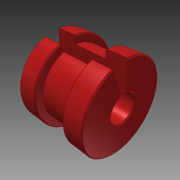
# Autodesk Inventor part: coupling_tie
Saved by Autodesk Inventor 2014 (Build 180170000, 170)
## iProperties
Created: 2014-01-25
Part Number: coupling_tie
Material: ABS Plastic
Document SubType Name: Modeling
Designer: buben
Density: 1.06 g/cm^3
Appearance: Light Red
Author: buben
Autodesk Inventor part; units mm, degrees
ref_plane "YZ Plane" through (0, 0, 0) normal (1, 0, 0) x (0, 1, 0)
ref_plane "XZ Plane" through (0, 0, 0) normal (0, 1, 0) x (-1, 0, 0)
ref_plane "XY Plane" through (0, 0, 0) normal (0, 0, 1) x (1, 0, 0)
sketch "Sketch1" plane through (0, 0, 0) normal (0, 1, 0) x (-1, 0, 0)
  line L0 (-9, 0) -> (9, 0)
  line L1 (-9, 3.5) -> (9, 3.5)
  line L2 (9, 3.5) -> (9, 11)
  line L3 (9, 11) -> (4, 11)
  line L4 (4, 11) -> (4, 9)
  line L5 (4, 9) -> (-4, 9)
  line L6 (-4, 9) -> (-4, 11)
  line L7 (-4, 11) -> (-9, 11)
  line L8 (-9, 11) -> (-9, 3.5)
  point P0 (0, 0)
  point P1 (0, 9)
  point P2 (0, 3.5)
  dimension "d0" = 18
  dimension "d1" = 8
  dimension "d2" = 7
  dimension "d3" = 22
  dimension "d4" = 2
  constraints: 18 end point, 7 parallel, 4 vertical alignment, 3 midpoint, 1 collinear, 1 horizontal, 1 perpendicular
  measures "d0" distance of L1.start L1.end
  measures "d1" distance of L4.end L5.end
  measures "d2" diameter of L1 L0
  measures "d3" diameter of L3 L0
  measures "d4" distance between parallel lines of L3 L5
revolve "Revolution1" add sketch "Sketch1" angle 340 about axis through (9, 0, 0) along (-1, 0, 0)
chamfer "Chamfer1" distance 0.3 angle 45 6 edges at (-4, 1.9101, -10.8329) (4, 1.9101, -10.8329) (9, 1.9101, -10.8329) (-9, 1.9101, -10.8329) (9, 0.6078, -3.4468) (-9, 0.6078, -3.4468)
body "Solid1"
